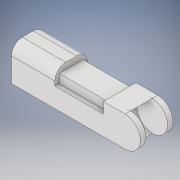
# Autodesk Inventor part: Part5
Saved by Autodesk Inventor 2017 SP1 (Build 210196100, 196)
## iProperties
Created: 2017-05-11
Part Number: Part5
Material: ABS Plastic
Document SubType Name: Modeling
Designer: zallen
Density: 1.06 g/cm^3
Appearance: Smooth - White
Author: zallen
Autodesk Inventor part; units mm, degrees
ref_plane "YZ Plane" through (0, 0, 0) normal (1, 0, 0) x (0, 1, 0)
ref_plane "XZ Plane" through (0, 0, 0) normal (0, 1, 0) x (-1, 0, 0)
sketch "Sketch1" plane through (0, 0, 0) normal (0, 0, 1) x (1, 0, 0)
  line L0 (0, 0) -> (0, 37.8188) construction
  line L1 (0, 0) -> (95.7615, 0) construction
  line L2 (0, 0) -> (261.6228, 0)
  line L3 (0, 0) -> (0, 70)
  arc A0 (261.6228, 0) -> (261.6228, 70) centre (261.6228, 35) ccw
  line L4 (261.6228, 70) -> (0, 70)
  dimension "d10" = 35
  constraints: 10 end point, 2 horizontal, 2 point on circle, 2 point on line, 1 centre point, 1 tangent, 1 vertical, 1 vertical alignment
  measures "d10" radius of A0
extrude "Extrusion1" add sketch "Sketch1" along normal mid plane 75
sketch "Sketch2" plane through (0, 0, 37.5) normal (-1, 0, 0) x (0, 0, 1)
  circle A0 centre (-37.5, 35) radius 12.5
  line L0 (0, 70) -> (0, 0) projected
  line L1 (0, 0) -> (-75, 0) projected
  point P0 (-37.5, 0)
  point P1 (-37.5, 0)
  dimension "d12" = 25
  dimension "d13" = 35
  constraints: 1 centre point, 1 midpoint, 1 vertical alignment
  measures "d12" diameter of A0
  measures "d13" distance of point (-37.5, 0) A0.centre
extrude "Extrusion2" add sketch "Sketch2" along normal blind 10
ref_plane "Work Plane1" through (0, 0, 0) normal (0, 0, -1) x (-1, 0, 0)
sketch "Sketch3" plane through (0, 0, 0) normal (0, 0, -1) x (-1, 0, 0)
  circle A0 centre (-261.6228, 35) radius 35
  arc A1 (-261.6228, 70) -> (-261.6228, 0) centre (-261.6228, 35) ccw projected
  point P0 (0, 0)
  dimension "d18" = 70
  constraints: 1 centre point, 1 concentric
  measures "d18" diameter of A0
extrude "Extrusion3" cut sketch "Sketch3" along normal mid plane 50
sketch "Sketch4" plane through (0, 0, 37.5) normal (0, 0, 1) x (1, 0, 0)
  line L0 (0, 70) -> (0, 0) projected
  line L1 (0, 70) -> (100, 70)
  line L2 (100, 70) -> (100, 80)
  line L3 (100, 80) -> (0, 80)
  line L4 (0, 80) -> (0, 70)
  dimension "d21" = 100
  dimension "d22" = 10
  constraints: 8 end point, 2 parallel, 1 horizontal, 1 perpendicular
  measures "d21" distance of L3.end L2.end
  measures "d22" distance of L2.end L1.end
extrude "Extrusion4" add sketch "Sketch4" against normal blind 75
sketch "Sketch5" plane through (0, 0, 37.5) normal (0, 0, 1) x (1, 0, 0)
  line L0 (261.6228, 70) -> (100, 70) projected
  line L1 (100, 70) -> (211.6228, 70)
  line L2 (211.6228, 70) -> (211.6228, 45)
  line L3 (211.6228, 45) -> (100, 45)
  line L4 (100, 45) -> (100, 70)
  point P0 (0, 0)
  dimension "d25" = 25
  dimension "d28" = 50
  constraints: 8 end point, 2 parallel, 1 horizontal
  measures "d25" distance of L1.end L2.end
  measures "d28" distance from line of L0.start L2
extrude "Extrusion5" cut sketch "Sketch5" against normal blind 10
sketch "Sketch6" plane through (0, 0, -37.5) normal (0, 0, -1) x (-1, 0, 0)
  line L0 (-100, 70) -> (-261.6228, 70) projected
  line L1 (-211.6228, 45) -> (-100, 45) projected
  line L2 (-100, 70) -> (-211.6228, 70)
  line L3 (-211.6228, 70) -> (-211.6228, 45)
  line L4 (-211.6228, 45) -> (-100, 45)
  line L5 (-100, 45) -> (-100, 70)
  point P0 (0, 0)
  constraints: 8 end point, 2 parallel, 1 horizontal, 1 perpendicular
extrude "Extrusion6" cut sketch "Sketch6" against normal blind 10
sketch "Sketch7" plane through (261.6228, 70, 25) normal (0, 1, 0) x (1, 0, 0)
  line L0 (-161.6228, -12.5) -> (-161.6228, 62.5) projected
  line L1 (-50, 52.5) -> (-161.6228, 52.5) projected
  line L2 (-161.6228, -2.5647) -> (-50, -2.5647)
  line L3 (-50, -2.5647) -> (-50, 52.5)
  line L4 (-50, 52.5) -> (-161.6228, 52.5)
  line L5 (-161.6228, 52.5) -> (-161.6228, -2.5647)
  point P0 (-261.6228, 25)
  constraints: 8 end point, 2 parallel, 1 horizontal, 1 perpendicular, 1 point on line
extrude "Extrusion7" cut sketch "Sketch7" against normal blind 5
fillet "Fillet1" radius 25 2 edges at (50, 80, 37.5) (50, 80, -37.5)
body "Solid1"
